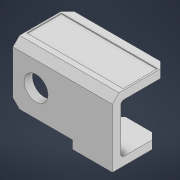
# Autodesk Inventor part: GF1002 mount
Saved by Autodesk Inventor 2021 (Build 250183000, 183)
## iProperties
Created: 2021-06-28
Part Number: GF1002 mount
Material: Generic
Document SubType Name: Modeling
Designer: allen
Density: 1 g/cm^3
Appearance: Default
Author: allen
Autodesk Inventor part; units mm, degrees
ref_plane "YZ Plane" through (0, 0, 0) normal (1, 0, 0) x (0, 1, 0)
ref_plane "XZ Plane" through (0, 0, 0) normal (0, 1, 0) x (-1, 0, 0)
ref_plane "XY Plane" through (0, 0, 0) normal (0, 0, 1) x (1, 0, 0)
sketch "Sketch1" plane through (0, 0, 0) normal (0, 0, 1) x (1, 0, 0)
  line L0 (0, 0) -> (30, 0)
  line L1 (30, 0) -> (30, 17.3)
  line L2 (30, 17.3) -> (0, 17.3)
  line L3 (0, 17.3) -> (0, 0)
  dimension "d0" = 30
  dimension "d1" = 17.3
  constraints: 8 end point, 2 parallel, 1 horizontal, 1 perpendicular
  measures "d0" distance of L0.start L0.end
  measures "d1" distance of L2.end L0.start
extrude "Extrusion1" add sketch "Sketch1" along normal blind 2.5
sketch "Sketch2" plane through (0, 0, 2.5) normal (0, 0, 1) x (1, 0, 0)
  line L0 (0, 17.3) -> (0, 0) projected
  line L1 (0, 0) -> (30, 0) projected
  point P0 (7, 8)
  dimension "d4" = 7
  dimension "d12" = 8
  measures "d4" distance from line of L0 point (7, 8)
  measures "d12" distance from line of point (7, 8) L1
hole "Hole1" at (7, 8, 2.5) direction (0, 0, -1) diameter 7.2 end through all
sketch "Sketch3" plane through (0, 0, 2.5) normal (0, 0, 1) x (1, 0, 0)
  line L0 (30, 0) -> (30, 17.3) projected
  line L1 (30, 0) -> (18, 0)
  line L2 (18, 0) -> (18, -2.5)
  line L3 (18, -2.5) -> (30, -2.5)
  line L4 (30, -2.5) -> (30, 0)
  point P0 (0, 0)
  dimension "d13" = 2.5
  dimension "d14" = 12
  constraints: 8 end point, 2 parallel, 1 horizontal, 1 perpendicular
  measures "d13" distance of L3.end L0.start
  measures "d14" distance of L2.end L3.end
extrude "Extrusion2" add sketch "Sketch3" against normal blind 14
sketch "Sketch4" plane through (18, 0, 0) normal (0, 1, 0) x (1, 0, 0)
  line L0 (3.25, 3) -> (8.75, 3)
  line L1 (8.75, 3) -> (8.75, 8.5)
  line L2 (8.75, 8.5) -> (3.25, 8.5)
  line L3 (3.25, 8.5) -> (3.25, 3)
  line L4 (0, 0) -> (0, 11.5) projected
  line L5 (0, 11.5) -> (12, 11.5) projected
  point P0 (-18, 0)
  point P1 (3.25, 5.75)
  point P2 (0, 5.75)
  point P3 (6, 8.5)
  point P4 (6, 11.5)
  dimension "d17" = 5.5
  constraints: 8 end point, 4 midpoint, 2 parallel, 2 perpendicular, 1 horizontal, 1 horizontal alignment, 1 vertical alignment
  measures "d17" distance of L1.end L2.end
extrude "Extrusion3" [suppressed]
fillet "Fillet1" [suppressed]
fillet "Fillet2" [suppressed]
fillet "Fillet3" radius 1 1 edges at (24, 0, 0)
sketch "Sketch5" plane through (0, 0, 0) normal (0, 0, -1) x (-1, 0, 0)
  line L0 (-30, 17.3) -> (0, 17.3) projected
  line L1 (-30, 1) -> (-30, 17.3) projected
  line L2 (0, 17.3) -> (0, 0) projected
  line L3 (-30, -2.5) -> (-30, 17.3) projected
  line L4 (0, 14.8) -> (-30, 14.8)
  point P0 (0, 2)
  dimension "d26" = 2.5
  constraints: 2 end point, 2 point on line
  measures "d26" distance between parallel lines of L0 L4
extrude "Extrusion4" add sketch "Sketch5" along normal blind 14
chamfer "Chamfer2" distance 2 angle 45 6 edges at (0, 0, 1.25) (18, -1.25, -11.5) (0, 16.05, -14) (30, 16.05, -14) (15, 17.3, 2.5) (30, -1.25, -11.5)
fillet "Fillet4" radius 1 1 edges at (15, 14.8, 0)
sketch "Sketch6" plane through (0, 17.3, 0.5) normal (0, 1, 0) x (1, 0, 0)
  line L0 (29.5, 12.1) -> (0.5, 12.1)
  line L1 (0.5, 12.1) -> (0.5, 1.7)
  line L2 (0.5, 1.7) -> (29.5, 1.7)
  line L3 (29.5, 1.7) -> (29.5, 12.1)
  line L4 (0, 12.5) -> (0, 0) projected
  line L5 (30, 12.5) -> (30, 0) projected
  line L6 (2, 14.5) -> (28, 14.5) projected
  point P0 (0, 0.5)
  dimension "d33" = 10.4
  dimension "d34" = 0.5
  dimension "d36" = 0.5
  dimension "d37" = 2.4
  constraints: 8 end point, 2 parallel, 1 horizontal, 1 perpendicular
  measures "d33" distance of L0.end L1.end
  measures "d34" distance between parallel lines of L4 L1
  measures "d36" distance between parallel lines of L5 L3
  measures "d37" distance between parallel lines of L6 L0
emboss "Emboss1" sketch "Sketch6" operation cut depth 0.2 direction (0, -1, 0)
body "Solid1"
